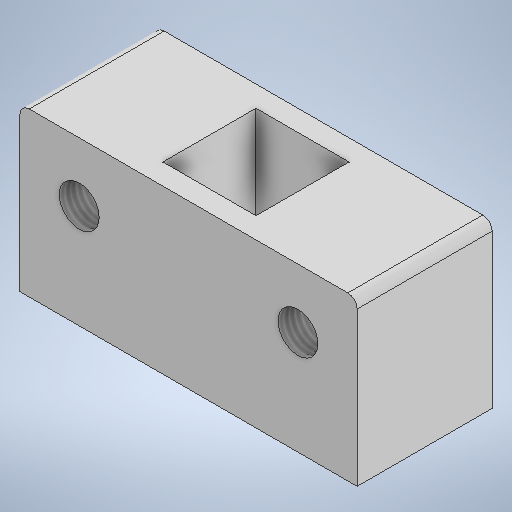
# Autodesk Inventor part: project_rough_mover
Saved by Autodesk Inventor 2025 (Build 290162000, 162)
## iProperties
Created: 2025-09-01
Part Number: project_rough_mover
Material: Generic
Document SubType Name: Modeling
Designer: Kiran
Density: 1 g/cm^3
Appearance: Default
Author: Kiran
Autodesk Inventor part; units mm, degrees
ref_plane "YZ Plane" through (0, 0, 0) normal (1, 0, 0) x (0, 1, 0)
ref_plane "XZ Plane" through (0, 0, 0) normal (0, 1, 0) x (-1, 0, 0)
ref_plane "XY Plane" through (0, 0, 0) normal (0, 0, 1) x (1, 0, 0)
sketch "Sketch1" plane through (0, 0, 0) normal (0, 0, 1) x (1, 0, 0)
  line L0 (130.1382, 2) -> (130.1382, 24.0208)
  line L1 (114.1591, 40) -> (3.1591, 40)
  line L2 (1.1591, -30) -> (130.1382, -30)
  line L3 (130.1382, -30) -> (130.1382, 2)
  line L4 (1.1591, -30) -> (-14.8135, -30)
  line L5 (-14.8135, -30) -> (-14.8135, 37.6368)
  line L6 (114.1591, 40) -> (126.1382, 40)
  line L7 (130.1382, 36) -> (130.1382, 24.0208)
  line L8 (126.1382, 40) -> (126.1382, 40)
  line L9 (130.1382, 36) -> (130.1382, 36)
  line L10 (-14.8135, 37.6368) -> (-14.8135, 36)
  line L11 (-10.8135, 40) -> (3.1591, 40)
  arc A0 (-10.8135, 40) -> (-14.8135, 36) centre (-10.8135, 36) ccw
  arc A1 (130.1382, 36) -> (126.1382, 40) centre (126.1382, 36) ccw
  circle A2 centre (104.5, 18) radius 8.6
  circle A3 centre (10.5, 18) radius 8.6
  point P0 (130.1382, 40)
  point P1 (-14.8135, 40)
  dimension "d41" = 4
  constraints: 24 end point, 5 point on line, 4 centre point, 4 perpendicular, 4 point on circle, 4 tangent, 2 collinear, 2 horizontal, 1 equal radius, 1 vertical
  measures "d41" radius of A0
extrude "Extrusion1" add sketch "Sketch1" along normal blind 58 contours L3 L2 L4 L5 A0 L11 L1 L6 A1 L7 L0 | A2 | A3
sketch "Sketch3" plane through (0, 0, 58) normal (0, 0, 1) x (1, 0, 0)
  circle A0 centre (104.5, 18) radius 10.5 projected
  circle A1 centre (10.495, 18) radius 10.5
  point P0 (0, 0)
  dimension "d28" = 21
  constraints: 1 centre point
  measures "d28" diameter of A1
extrude "Extrusion3" cut sketch "Sketch3" against normal blind 90 contours A1
sketch "Sketch4" plane through (-14.8135, 40, 0) normal (0, 1, 0) x (1, 0, 0)
  line L0 (52.4758, -29) -> (52.4758, -9)
  line L1 (52.4758, -9) -> (72.4758, -9)
  line L2 (52.4758, -9) -> (92.4758, -9)
  line L3 (92.4758, -9) -> (92.4758, -49)
  line L4 (92.4758, -49) -> (52.4758, -49)
  line L5 (52.4758, -49) -> (52.4758, -9)
  point P0 (14.8135, 0)
  dimension "d31" = 20
  dimension "d32" = 20
  dimension "d33" = 40
  dimension "d34" = 40
  constraints: 12 end point, 2 parallel, 1 horizontal, 1 perpendicular
  measures "d31" distance of L0.end L1.end
  measures "d32" distance of L0.start L0.end
  measures "d33" distance of L3.end L4.end
  measures "d34" distance of L2.end L3.end
extrude "Extrusion4" cut sketch "Sketch4" against normal blind 70
sketch "Sketch5" plane through (0, 0, 0) normal (0, 0, -1) x (-1, 0, 0)
  point P0 (0, 0)
sketch "Sketch6" plane through (0, 0, 58) normal (0, 0, 1) x (1, 0, 0)
  circle A0 centre (10.495, 18) radius 10.5 projected
  circle A1 centre (10.495, 18) radius 10.5
  point P0 (0, 0)
  constraints: 1 centre point, 1 coincident
extrude "Extrusion5" add sketch "Sketch6" against normal blind 58
sketch "Sketch7" plane through (0, 0, 58) normal (0, 0, 1) x (1, 0, 0)
  line L0 (-14.8135, 36) -> (-14.8135, -30) projected
  line L1 (130.1382, -30) -> (130.1382, 36) projected
  line L2 (-14.8135, 14.5974) -> (130.1865, 14.5974)
  line L3 (57.6865, 14.5974) -> (10.684, 14.5974)
  line L4 (10.684, 14.5974) -> (104.689, 14.5974)
  circle A0 centre (104.689, 14.5974) radius 8.6
  circle A1 centre (10.684, 14.5974) radius 8.6
  point P0 (0, 0)
  dimension "d48" = 47.0025
  dimension "d49" = 94.005
  dimension "d50" = 17.2
  dimension "d51" = 17.2
  constraints: 6 end point, 3 point on line, 2 centre point, 2 coincident, 1 midpoint, 1 perpendicular
  measures "d48" distance of L3.start L3.end
  measures "d49" distance of L3.end L4.end
  measures "d50" diameter of A0
  measures "d51" diameter of A1
extrude "Extrusion6" cut sketch "Sketch7" against normal blind 58
thread "Thread5" size "M18x2.5" class "6H" standard "ANSI Metric M Profile" full length
thread "Thread6" size "M18x2.5" class "6H" standard "ANSI Metric M Profile" full length
body "Solid1"
